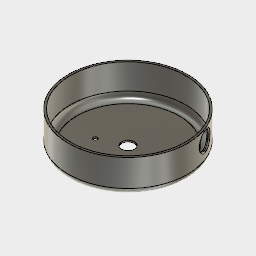
TelepresenceBase (Autodesk Fusion 360 design; units mm, degrees)
Autodesk Fusion 360 part; units mm, degrees
sketch "Sketch1" plane through (0, 0, 0) normal (0, 0, 1) x (1, 0, 0)
  circle A0 centre (0, 0) radius 45
  circle A1 centre (0, 0) radius 5
  line L0 (0, 45) -> (0, -45) construction
  line L1 (-45, 0) -> (45, 0) construction
  line L2 (-17.5, -8) -> (17.5, -8) construction
  circle A2 centre (-17.5, -8) radius 1.6
  circle A3 centre (17.5, -8) radius 1.6
  circle A4 centre (0, 0) radius 46.6
  point P0 (0, -8)
  dimension "d1" = 90
  dimension "d2" = 10
  dimension "d3" = 8
  dimension "d4" = 35
  dimension "d5" = 3.2
  dimension "d6" = 3.2
  dimension "d9" = 1.6
  measures "d1" diameter of A0
  measures "d2" diameter of A1
  measures "d3" distance of L1 L2
  measures "d4" distance of L2.start L2.end
  measures "d5" diameter of A2
  measures "d6" diameter of A3
extrude "Extrude1" add sketch "Sketch1" along normal blind 1.2 contours A0
extrude "Extrude2" add sketch "Sketch1" along normal blind 26 contours A4
fillet "Fillet1" radius 5 1 edges at (-41.9547, -16.2727, 1.2)
fillet "Fillet2" radius 5 1 edges at (-43.4465, -16.8513, 0)
ref_plane "WorkPlane1" through (43.2454, 17.3608, 15.1482) normal (0.928012, 0.37255, 0) x (0.37255, -0.928012, 0)
sketch "Sketch2" plane through (43.2454, 17.3608, 15.1482) normal (0.928012, 0.37255, 0) x (0.37255, -0.928012, 0)
  circle A0 centre (0, -2.1018) radius 6.75
  line L0 (-46.6, -10.8518) -> (46.6, -10.8518)
  dimension "d15" = 13.5
  dimension "d16" = 8.75
  measures "d15" diameter of A0
  measures "d16" distance of A0.centre L0
extrude "Extrude3" cut sketch "Sketch2" against normal blind 5
fillet "Fillet3" radius 0.75 2 edges at (40.2746, 23.4418, 17.25) (45.304, 10.9137, 17.25)
equation "d6 = d5"
equation "d16 = d15 / 2 + 2 mm"
named bodies: "PhoneBase"
